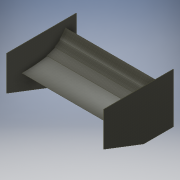
# Autodesk Inventor part: R-wing
Saved by Autodesk Inventor 2018.1 (Build 221171000, 171)
## iProperties
Created: 2017-10-11
Part Number: R-wing
Material: PAEK 樹脂
Document SubType Name: Modeling
Designer: kuwano
Density: 1.32 g/cm^3
Appearance: カーボンファイバー 1
Author: kuwano
Autodesk Inventor part; units mm, degrees
ref_plane "YZ Plane" through (0, 0, 0) normal (1, 0, 0) x (0, 1, 0)
ref_plane "XZ Plane" through (0, 0, 0) normal (0, 1, 0) x (-1, 0, 0)
ref_plane "XY Plane" through (0, 0, 0) normal (0, 0, 1) x (1, 0, 0)
sketch "スケッチ1" plane through (0, 0, 0) normal (1, 0, 0) x (0, 1, 0)
  arc A0 (0, 250) -> (23.6219, -20) centre (550.3346, 162.1147) ccw
  arc A1 (0, 250) -> (23.6219, -20) centre (1554.868, 250) ccw
  line L0 (0, 250) -> (23.6219, -20)
  line L1 (0, -286.5226) -> (0, 339.4204) projected
  line L2 (-330.9698, 0) -> (1869.1743, 0) projected
  arc A2 (26.8913, 0) -> (63.2883, -100) centre (478.3817, 107.7054) ccw
  arc A3 (26.8913, 0) -> (63.2883, -100) centre (174.3048, -2.9696) ccw
  line L3 (26.8913, 0) -> (63.2883, -100)
  arc A4 (61.3298, -80) -> (110.3443, -150) centre (417.9077, 117.5184) ccw
  arc A5 (61.3298, -80) -> (110.3443, -150) centre (163.7866, -60.4191) ccw
  line L4 (61.3298, -80) -> (110.3443, -150)
  arc A6 (102.444, -130) -> (173.9492, -190) centre (412.3652, 166.7414) ccw
  arc A7 (102.444, -130) -> (173.9492, -190) centre (210.7273, -73.5613) ccw
  line L5 (102.444, -130) -> (173.9492, -190)
  dimension "d14" = 5
  dimension "d15" = 250
  dimension "d18" = 15
  dimension "d19" = 20
  dimension "d20" = 100
  dimension "d21" = 270
  dimension "d22" = 15
  dimension "d23" = 20
  dimension "d24" = 5
  dimension "d25" = 5
  dimension "d26" = 70
  dimension "d37" = 15
  dimension "d38" = 20
  dimension "d39" = 5
  dimension "d40" = 60
  constraints: 16 point on circle, 8 centre point, 8 end point, 4 tangent, 1 point on line
  measures "d14" angle of L1 L0
  measures "d15" distance from line of L2 L0.start
  measures "d18" angle of L3 L0
  measures "d19" vertical distance of L0.end L3.start
  measures "d20" vertical distance of L3.start L3.end
  measures "d21" vertical distance of L0.end L0.start
  measures "d22" angle of L4 L3
  measures "d23" vertical distance of L3.end L4.start
  measures "d24" distance from line of L0 L3.start
  measures "d25" distance from line of L3 L4.start
  measures "d26" vertical distance of L4.end L4.start
  measures "d37" angle of L4 L5
  measures "d38" vertical distance of L4.end L5.start
  measures "d39" distance from line of L4 L5.start
  measures "d40" vertical distance of L5.start L5.end
extrude "押し出し3" add sketch "スケッチ1" along normal mid plane 970 contours L1 A0 | A2 A3 | A1 L2 A0 L1 | A1 A0 L2 | A4 A5 | A6 A7
sketch "スケッチ3" plane through (485, 0, 0) normal (1, 0, 0) x (0, 0, -1)
  line L0 (-400, 246.344) -> (299.3328, 246.344)
  line L1 (299.3328, 246.344) -> (299.3328, -253.656)
  line L2 (299.3328, -253.656) -> (0, -253.656)
  line L3 (0, -253.656) -> (-400, -100)
  line L4 (-400, -100) -> (-400, 246.344)
  arc A0 (0, 26.8913) -> (100, 63.2883) centre (2.9696, 174.3048) ccw projected
  line L5 (0, 26.8913) -> (0, -253.656)
  point P0 (0, 0)
  point P1 (150, 110.3443)
  point P2 (-250, 0)
  dimension "d31" = 100
  dimension "d32" = 150
  dimension "d34" = 500
  constraints: 12 end point, 4 perpendicular, 1 horizontal
  measures "d31" vertical distance of L3.end point (-250, 0)
  measures "d32" horizontal distance of point (-250, 0) L3.end
  measures "d34" distance of L0.end L1.end
extrude "押し出し4" add sketch "スケッチ3" along normal blind 3
mirror "ミラー2" about plane through (0, 0, 0) normal (1, 0, 0) of "押し出し4"
